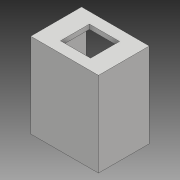
# Autodesk Inventor part: case
Saved by Autodesk Inventor 2017 (Build 210142000, 142)
## iProperties
Created: 2017-01-02
Part Number: case
Material: Generic
Document SubType Name: Modeling
Designer: Sachin Konan
Density: 1 g/cm^3
Appearance: Default
Author: Sachin Konan
Autodesk Inventor part; units mm, degrees
ref_plane "YZ Plane" through (0, 0, 0) normal (1, 0, 0) x (0, 1, 0)
ref_plane "XZ Plane" through (0, 0, 0) normal (0, 1, 0) x (-1, 0, 0)
ref_plane "XY Plane" through (0, 0, 0) normal (0, 0, 1) x (1, 0, 0)
sketch "Sketch1" plane through (0, 0, 0) normal (0, 1, 0) x (-1, 0, 0)
  line L0 (0, 0) -> (120, 0)
  line L1 (120, 0) -> (120, -150)
  line L2 (120, -150) -> (0, -150)
  line L3 (0, -150) -> (0, 0)
  dimension "d0" = 120
  dimension "d1" = 150
  constraints: 8 end point, 2 parallel, 1 horizontal, 1 perpendicular
  measures "d0" distance of L1.end L2.end
  measures "d1" distance of L0.end L1.end
extrude "Extrusion1" add sketch "Sketch1" along normal blind 90
shell "Shell1" thickness 8 removed faces 1 at (-80, 90, -100)
sketch "Sketch2" plane through (-120, 0, 0) normal (0, 0, 1) x (1, 0, 0)
  line L0 (120, 0) -> (0, 0) projected
  line L1 (0, 0) -> (0, 90) projected
  line L2 (86.681, 70.681) -> (33.319, 70.681)
  line L3 (33.319, 70.681) -> (33.319, 19.319)
  line L4 (33.319, 19.319) -> (86.681, 19.319)
  line L5 (86.681, 19.319) -> (86.681, 70.681)
  line L6 (86.681, 70.681) -> (33.319, 19.319) construction
  line L7 (33.319, 70.681) -> (86.681, 19.319) construction
  dimension "d5" = 53.362
  dimension "d6" = 51.362
  constraints: 12 end point, 2 parallel, 1 horizontal, 1 perpendicular
  measures "d5" distance of L4.end L3.end
  measures "d6" distance of L4.end L2.start
extrude "Extrusion2" cut sketch "Sketch2" against normal blind 80
body "Solid1"
